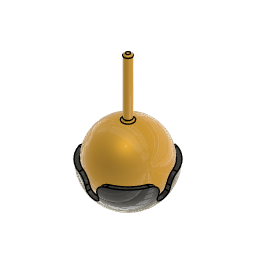
Ball Joint v1 (Autodesk Fusion 360 design; units mm, degrees)
Autodesk Fusion 360 part; units mm, degrees
note: some values were not read from the file. Set by a fixed rule: which sketch regions a step uses.
sketch "Sketch1" plane through (0, 0, 0) normal (0, 1, 0) x (1, 0, 0)
  circle A0 centre (0, 0) radius 5
  circle A1 centre (0, 0) radius 4.5
  line L0 (0, -8) -> (0, 7.2449)
  line L1 (7.5, 0) -> (-7.5, 0)
  line L2 (0, 0) -> (0.5, 0)
  line L3 (0.5, 0) -> (0.5, -12)
  line L4 (0.5, -12) -> (0, -12)
  line L5 (0, -12) -> (0, 0)
  dimension "d1" = 10
  dimension "d2" = 9
  dimension "d3" = 0.5
  dimension "d4" = 12
  constraint coincident A0.centre A1.centre
  constraint vertical L0
  constraint perpendicular L0 L1
  constraint horizontal L2
  constraint vertical L3
  constraint horizontal L4
  constraint vertical L5
  measures "d1" diameter of A0
  measures "d2" diameter of A1
  measures "d3" distance of A0.centre L2.end
  measures "d4" distance of A0.centre L4.end
revolve "Revolve1" add sketch "Sketch1" angle 360 about axis through (0, 0, 12) along (0, 0, -1) contours A0 A1 L0 L1 picked at (0.2372, 4.8164) makes body 1 in component "Component"
revolve "Revolve1'" add sketch "Sketch1" angle 360 about axis through (0, 0, 12) along (0, 0, -1) separate body contours A0 L0 L3 L4 L5 | A0 A1 L0 L3 L5 | A1 L0 L1 L2 | A1 L1 L3 | A1 L0 L1 L2 L3 L5 makes body 2 in component "Component'"
fillet "Fillet1" radius 0.25 2 edges at (-0.4662, -0.1808, 4.4721) (-0.4662, -0.1808, 12) on bodies 2 in component "Component'"
sketch "Sketch1 (2)" plane through (0, 0, 0) normal (0, 1, 0) x (1, 0, 0) in component "Component"
  line L0 (-0.75, 1.75) -> (-0.75, -2.5)
  line L1 (-0.75, -2.5) -> (0.75, -2.5)
  line L2 (0.75, -2.5) -> (0.75, 1.75)
  line L3 (0.75, 2.5) -> (-0.75, -2.5) construction
  line L4 (-0.75, 2.5) -> (0.75, -2.5) construction
  arc A0 (0, 2.5) -> (-0.75, 1.75) centre (0, 1.75) ccw
  arc A1 (0.75, 1.75) -> (0, 2.5) centre (0, 1.75) ccw
  dimension "d9" = 1.5
  dimension "d10" = 5
  dimension "d11" = 0.75
  constraint parallel L0 L2
  constraint coincident L3 origin
  constraint coincident L4 origin
  constraint coincident L4.start L0
  constraint tangent L0 A0
  constraint coincident L3.start L2
  constraint tangent L2 A1
  constraint equal A0 A1
  constraint coincident A0.start A1.end
  measures "d9" distance of L0.end L1.end
  measures "d10" distance of L4.start L0.end
  measures "d11" radius of A0
extrude "Extrude1" cut sketch "Sketch1 (2)" along normal blind 6 bodies 1 in component "Component"
fillet "Fillet1'" radius 1 2 edges at (0.75, 4.6902, 0) (-0.75, 4.6902, 0) on bodies 1 in component "Component"
pattern_circular "C-Pattern1" count 4 over 360 about axis through (0, 0, 1.75) along (0, 0, 1) of "Extrude1", "Fillet1'" in component "Component"
component "Component" placed x (1, 0, 0) y (0, 1, 0) z (0, 0, 1) at (0, 0, 0)
component "Component'" placed x (1, 0, 0) y (0, 1, 0) z (0, 0, 1) at (0, 0, 0)
